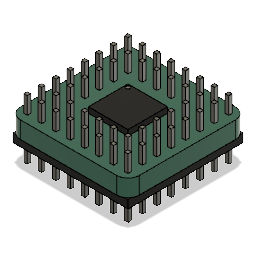
PGA2040 (Autodesk Fusion 360 design; units mm, degrees)
Autodesk Fusion 360 part; units mm, degrees
note: some values were not read from the file. Set by a fixed rule: which sketch regions a step uses.
sketch "Sketch1" plane through (0, 0, 0) normal (0, 1, 0) x (1, 0, 0)
  line L0 (-10.5, 10.5) -> (10.5, 10.5)
  line L1 (10.5, 10.5) -> (10.5, -10.5)
  line L2 (10.5, -10.5) -> (-10.5, -10.5)
  line L3 (-10.5, -10.5) -> (-10.5, 10.5)
  line L4 (-3.5, 3.5) -> (3.5, 3.5)
  line L5 (3.5, 3.5) -> (3.5, -3.5)
  line L6 (3.5, -3.5) -> (-3.5, -3.5)
  line L7 (-3.5, -3.5) -> (-3.5, 3.5)
  line L8 (-10.5, 8.89) -> (10.5, 8.89) construction
  line L9 (-8.89, 10.5) -> (-8.89, -10.5) construction
  line L10 (-10.5, -8.89) -> (10.5, -8.89) construction
  line L11 (8.89, 10.5) -> (8.89, -10.5) construction
  line L12 (-8.57, 8.57) -> (-9.21, 8.57)
  line L13 (-9.21, 8.57) -> (-9.21, 9.21)
  line L14 (-9.21, 9.21) -> (-8.57, 9.21)
  line L15 (-8.57, 9.21) -> (-8.57, 8.57)
  line L16 (-8.57, 8.57) -> (-9.21, 9.21) construction
  line L17 (-9.21, 8.57) -> (-8.57, 9.21) construction
  line L18 (-6.67, 9.21) -> (-6.03, 9.21)
  line L19 (-6.67, 8.57) -> (-6.67, 9.21)
  line L20 (-6.03, 8.57) -> (-6.67, 8.57)
  line L21 (-6.03, 9.21) -> (-6.03, 8.57)
  line L22 (-4.13, 9.21) -> (-3.49, 9.21)
  line L23 (-4.13, 8.57) -> (-4.13, 9.21)
  line L24 (-3.49, 8.57) -> (-4.13, 8.57)
  line L25 (-3.49, 9.21) -> (-3.49, 8.57)
  line L26 (-1.59, 9.21) -> (-0.95, 9.21)
  line L27 (-1.59, 8.57) -> (-1.59, 9.21)
  line L28 (-0.95, 8.57) -> (-1.59, 8.57)
  line L29 (-0.95, 9.21) -> (-0.95, 8.57)
  line L30 (0.95, 9.21) -> (1.59, 9.21)
  line L31 (0.95, 8.57) -> (0.95, 9.21)
  line L32 (1.59, 8.57) -> (0.95, 8.57)
  line L33 (1.59, 9.21) -> (1.59, 8.57)
  line L34 (3.49, 9.21) -> (4.13, 9.21)
  line L35 (3.49, 8.57) -> (3.49, 9.21)
  line L36 (4.13, 8.57) -> (3.49, 8.57)
  line L37 (4.13, 9.21) -> (4.13, 8.57)
  line L38 (6.03, 9.21) -> (6.67, 9.21)
  line L39 (6.03, 8.57) -> (6.03, 9.21)
  line L40 (6.67, 8.57) -> (6.03, 8.57)
  line L41 (6.67, 9.21) -> (6.67, 8.57)
  line L42 (8.57, 9.21) -> (9.21, 9.21)
  line L43 (8.57, 8.57) -> (8.57, 9.21)
  line L44 (9.21, 8.57) -> (8.57, 8.57)
  line L45 (9.21, 9.21) -> (9.21, 8.57)
  line L46 (-9.21, 6.67) -> (-8.57, 6.67)
  line L47 (-9.21, 6.03) -> (-9.21, 6.67)
  line L48 (-8.57, 6.03) -> (-9.21, 6.03)
  line L49 (-8.57, 6.67) -> (-8.57, 6.03)
  line L50 (-6.67, 6.67) -> (-6.03, 6.67)
  line L51 (-6.67, 6.03) -> (-6.67, 6.67)
  line L52 (-6.03, 6.03) -> (-6.67, 6.03)
  line L53 (-6.03, 6.67) -> (-6.03, 6.03)
  line L54 (-4.13, 6.67) -> (-3.49, 6.67)
  line L55 (-4.13, 6.03) -> (-4.13, 6.67)
  line L56 (-3.49, 6.03) -> (-4.13, 6.03)
  line L57 (-3.49, 6.67) -> (-3.49, 6.03)
  line L58 (-1.59, 6.67) -> (-0.95, 6.67)
  line L59 (-1.59, 6.03) -> (-1.59, 6.67)
  line L60 (-0.95, 6.03) -> (-1.59, 6.03)
  line L61 (-0.95, 6.67) -> (-0.95, 6.03)
  line L62 (0.95, 6.67) -> (1.59, 6.67)
  line L63 (0.95, 6.03) -> (0.95, 6.67)
  line L64 (1.59, 6.03) -> (0.95, 6.03)
  line L65 (1.59, 6.67) -> (1.59, 6.03)
  line L66 (3.49, 6.67) -> (4.13, 6.67)
  line L67 (3.49, 6.03) -> (3.49, 6.67)
  line L68 (4.13, 6.03) -> (3.49, 6.03)
  line L69 (4.13, 6.67) -> (4.13, 6.03)
  line L70 (6.03, 6.67) -> (6.67, 6.67)
  line L71 (6.03, 6.03) -> (6.03, 6.67)
  line L72 (6.67, 6.03) -> (6.03, 6.03)
  line L73 (6.67, 6.67) -> (6.67, 6.03)
  line L74 (8.57, 6.67) -> (9.21, 6.67)
  line L75 (8.57, 6.03) -> (8.57, 6.67)
  line L76 (9.21, 6.03) -> (8.57, 6.03)
  line L77 (9.21, 6.67) -> (9.21, 6.03)
  line L78 (-9.21, 4.13) -> (-8.57, 4.13)
  line L79 (-9.21, 3.49) -> (-9.21, 4.13)
  line L80 (-8.57, 3.49) -> (-9.21, 3.49)
  line L81 (-8.57, 4.13) -> (-8.57, 3.49)
  line L82 (-6.67, 4.13) -> (-6.03, 4.13)
  line L83 (-6.67, 3.49) -> (-6.67, 4.13)
  line L84 (-6.03, 3.49) -> (-6.67, 3.49)
  line L85 (-6.03, 4.13) -> (-6.03, 3.49)
  line L86 (6.03, 4.13) -> (6.67, 4.13)
  line L87 (6.03, 3.49) -> (6.03, 4.13)
  line L88 (6.67, 3.49) -> (6.03, 3.49)
  line L89 (6.67, 4.13) -> (6.67, 3.49)
  line L90 (8.57, 4.13) -> (9.21, 4.13)
  line L91 (8.57, 3.49) -> (8.57, 4.13)
  line L92 (9.21, 3.49) -> (8.57, 3.49)
  line L93 (9.21, 4.13) -> (9.21, 3.49)
  line L94 (-9.21, 1.59) -> (-8.57, 1.59)
  line L95 (-9.21, 0.95) -> (-9.21, 1.59)
  line L96 (-8.57, 0.95) -> (-9.21, 0.95)
  line L97 (-8.57, 1.59) -> (-8.57, 0.95)
  line L98 (-6.67, 1.59) -> (-6.03, 1.59)
  line L99 (-6.67, 0.95) -> (-6.67, 1.59)
  line L100 (-6.03, 0.95) -> (-6.67, 0.95)
  line L101 (-6.03, 1.59) -> (-6.03, 0.95)
  line L102 (6.03, 1.59) -> (6.67, 1.59)
  line L103 (6.03, 0.95) -> (6.03, 1.59)
  line L104 (6.67, 0.95) -> (6.03, 0.95)
  line L105 (6.67, 1.59) -> (6.67, 0.95)
  line L106 (8.57, 1.59) -> (9.21, 1.59)
  line L107 (8.57, 0.95) -> (8.57, 1.59)
  line L108 (9.21, 0.95) -> (8.57, 0.95)
  line L109 (9.21, 1.59) -> (9.21, 0.95)
  line L110 (-9.21, -0.95) -> (-8.57, -0.95)
  line L111 (-9.21, -1.59) -> (-9.21, -0.95)
  line L112 (-8.57, -1.59) -> (-9.21, -1.59)
  line L113 (-8.57, -0.95) -> (-8.57, -1.59)
  line L114 (-6.67, -0.95) -> (-6.03, -0.95)
  line L115 (-6.67, -1.59) -> (-6.67, -0.95)
  line L116 (-6.03, -1.59) -> (-6.67, -1.59)
  line L117 (-6.03, -0.95) -> (-6.03, -1.59)
  line L118 (6.03, -0.95) -> (6.67, -0.95)
  line L119 (6.03, -1.59) -> (6.03, -0.95)
  line L120 (6.67, -1.59) -> (6.03, -1.59)
  line L121 (6.67, -0.95) -> (6.67, -1.59)
  line L122 (8.57, -0.95) -> (9.21, -0.95)
  line L123 (8.57, -1.59) -> (8.57, -0.95)
  line L124 (9.21, -1.59) -> (8.57, -1.59)
  line L125 (9.21, -0.95) -> (9.21, -1.59)
  line L126 (-9.21, -3.49) -> (-8.57, -3.49)
  line L127 (-9.21, -4.13) -> (-9.21, -3.49)
  line L128 (-8.57, -4.13) -> (-9.21, -4.13)
  line L129 (-8.57, -3.49) -> (-8.57, -4.13)
  line L130 (-6.67, -3.49) -> (-6.03, -3.49)
  line L131 (-6.67, -4.13) -> (-6.67, -3.49)
  line L132 (-6.03, -4.13) -> (-6.67, -4.13)
  line L133 (-6.03, -3.49) -> (-6.03, -4.13)
  line L134 (6.03, -3.49) -> (6.67, -3.49)
  line L135 (6.03, -4.13) -> (6.03, -3.49)
  line L136 (6.67, -4.13) -> (6.03, -4.13)
  line L137 (6.67, -3.49) -> (6.67, -4.13)
  line L138 (8.57, -3.49) -> (9.21, -3.49)
  line L139 (8.57, -4.13) -> (8.57, -3.49)
  line L140 (9.21, -4.13) -> (8.57, -4.13)
  line L141 (9.21, -3.49) -> (9.21, -4.13)
  line L142 (-9.21, -6.03) -> (-8.57, -6.03)
  line L143 (-9.21, -6.67) -> (-9.21, -6.03)
  line L144 (-8.57, -6.67) -> (-9.21, -6.67)
  line L145 (-8.57, -6.03) -> (-8.57, -6.67)
  line L146 (-6.67, -6.03) -> (-6.03, -6.03)
  line L147 (-6.67, -6.67) -> (-6.67, -6.03)
  line L148 (-6.03, -6.67) -> (-6.67, -6.67)
  line L149 (-6.03, -6.03) -> (-6.03, -6.67)
  line L150 (-4.13, -6.03) -> (-3.49, -6.03)
  line L151 (-4.13, -6.67) -> (-4.13, -6.03)
  line L152 (-3.49, -6.67) -> (-4.13, -6.67)
  line L153 (-3.49, -6.03) -> (-3.49, -6.67)
  line L154 (-1.59, -6.03) -> (-0.95, -6.03)
  line L155 (-1.59, -6.67) -> (-1.59, -6.03)
  line L156 (-0.95, -6.67) -> (-1.59, -6.67)
  line L157 (-0.95, -6.03) -> (-0.95, -6.67)
  line L158 (0.95, -6.03) -> (1.59, -6.03)
  line L159 (0.95, -6.67) -> (0.95, -6.03)
  line L160 (1.59, -6.67) -> (0.95, -6.67)
  line L161 (1.59, -6.03) -> (1.59, -6.67)
  line L162 (3.49, -6.03) -> (4.13, -6.03)
  line L163 (3.49, -6.67) -> (3.49, -6.03)
  line L164 (4.13, -6.67) -> (3.49, -6.67)
  line L165 (4.13, -6.03) -> (4.13, -6.67)
  line L166 (6.03, -6.03) -> (6.67, -6.03)
  line L167 (6.03, -6.67) -> (6.03, -6.03)
  line L168 (6.67, -6.67) -> (6.03, -6.67)
  line L169 (6.67, -6.03) -> (6.67, -6.67)
  line L170 (8.57, -6.03) -> (9.21, -6.03)
  line L171 (8.57, -6.67) -> (8.57, -6.03)
  line L172 (9.21, -6.67) -> (8.57, -6.67)
  line L173 (9.21, -6.03) -> (9.21, -6.67)
  line L174 (-9.21, -8.57) -> (-8.57, -8.57)
  line L175 (-9.21, -9.21) -> (-9.21, -8.57)
  line L176 (-8.57, -9.21) -> (-9.21, -9.21)
  line L177 (-8.57, -8.57) -> (-8.57, -9.21)
  line L178 (-6.67, -8.57) -> (-6.03, -8.57)
  line L179 (-6.67, -9.21) -> (-6.67, -8.57)
  line L180 (-6.03, -9.21) -> (-6.67, -9.21)
  line L181 (-6.03, -8.57) -> (-6.03, -9.21)
  line L182 (-4.13, -8.57) -> (-3.49, -8.57)
  line L183 (-4.13, -9.21) -> (-4.13, -8.57)
  line L184 (-3.49, -9.21) -> (-4.13, -9.21)
  line L185 (-3.49, -8.57) -> (-3.49, -9.21)
  line L186 (-1.59, -8.57) -> (-0.95, -8.57)
  line L187 (-1.59, -9.21) -> (-1.59, -8.57)
  line L188 (-0.95, -9.21) -> (-1.59, -9.21)
  line L189 (-0.95, -8.57) -> (-0.95, -9.21)
  line L190 (0.95, -8.57) -> (1.59, -8.57)
  line L191 (0.95, -9.21) -> (0.95, -8.57)
  line L192 (1.59, -9.21) -> (0.95, -9.21)
  line L193 (1.59, -8.57) -> (1.59, -9.21)
  line L194 (3.49, -8.57) -> (4.13, -8.57)
  line L195 (3.49, -9.21) -> (3.49, -8.57)
  line L196 (4.13, -9.21) -> (3.49, -9.21)
  line L197 (4.13, -8.57) -> (4.13, -9.21)
  line L198 (6.03, -8.57) -> (6.67, -8.57)
  line L199 (6.03, -9.21) -> (6.03, -8.57)
  line L200 (6.67, -9.21) -> (6.03, -9.21)
  line L201 (6.67, -8.57) -> (6.67, -9.21)
  line L202 (8.57, -8.57) -> (9.21, -8.57)
  line L203 (8.57, -9.21) -> (8.57, -8.57)
  line L204 (9.21, -9.21) -> (8.57, -9.21)
  line L205 (9.21, -8.57) -> (9.21, -9.21)
  circle A0 centre (-3, 3) radius 0.375
  point P0 (-8.89, 8.89)
  dimension "d1" = 10.5
  dimension "d2" = 21
  dimension "d3" = 10.5
  dimension "d4" = 21
  dimension "d5" = 7
  dimension "d6" = 7
  dimension "d7" = 3.5
  dimension "d8" = 3.5
  dimension "d20" = 17.78
  dimension "d21" = 17.78
  dimension "d22" = 8.89
  dimension "d23" = 8.89
  dimension "d38" = 0.64
  dimension "d39" = 0.64
  dimension "d46" = 2.54
  dimension "d47" = -2.54
  dimension "d52" = 0.5
  dimension "d53" = 0.5
  dimension "d54" = 0.75
  constraint horizontal L0
  constraint vertical L1
  constraint horizontal L2
  constraint vertical L3
  constraint horizontal L4
  constraint vertical L5
  constraint horizontal L6
  constraint vertical L7
  constraint perpendicular L1 L8
  constraint coincident L1 L8.end
  constraint coincident L3 L8.start
  constraint perpendicular L2 L9
  constraint coincident L2 L9.end
  constraint coincident L0 L9.start
  constraint parallel L2 L10
  constraint coincident L1 L10.end
  constraint coincident L3 L10.start
  constraint perpendicular L2 L11
  constraint coincident L2 L11.end
  constraint coincident L0 L11.start
  constraint horizontal L12
  constraint perpendicular L12 L13
  constraint parallel L12 L14
  constraint parallel L13 L15
  constraint coincident L16 P0
  constraint coincident L17 P0
  constraint coincident L9 P0
  constraint coincident L8 P0
  measures "d1" distance of origin L0
  measures "d2" distance of L0 L2
  measures "d3" distance of origin L3
  measures "d4" distance of L1 L3
  measures "d5" distance of L4.start L4.end
  measures "d6" distance of L4.start L6.end
  measures "d7" distance of origin L4
  measures "d8" distance of origin L7
  measures "d20" distance of L9 L11
  measures "d21" distance of L8 L10
  measures "d22" distance of origin L10
  measures "d23" distance of origin L11
  measures "d38" distance of L13.end L14.end
  measures "d39" distance of L12.start L14.end
  measures "d52" distance of L7 A0.centre
  measures "d53" vertical distance of L4.start A0.centre
  measures "d54" diameter of A0
extrude "Extrude1" add sketch "Sketch1" along normal blind 1 contours L4 L5 L6 L7 | A0
extrude "Extrude2" add sketch "Sketch1" against normal blind 3 contours L0 L1 L2 L3 | L4 L5 L6 L7 | L12 L13 L14 L15 | L18 L19 L20 L21 | L22 L23 L24 L25 | L26 L27 L28 L29 | L30 L31 L32 L33 | L34 L35 L36 L37 | L38 L39 L40 L41 | L42 L43 L44 L45 | L46 L47 L48 L49 | L50 L51 L52 L53 | L54 L55 L56 L57 | L58 L59 L60 L61 | L62 L63 L64 L65 | L66 L67 L68 L69 | L70 L71 L72 L73 | L74 L75 L76 L77 | L78 L79 L80 L81 | L82 L83 L84 L85 | L86 L87 L88 L89 | L90 L91 L92 L93 | L94 L95 L96 L97 | L98 L99 L100 L101 | L102 L103 L104 L105 | L106 L107 L108 L109 | L110 L111 L112 L113 | L114 L115 L116 L117 | L118 L119 L120 L121 | L122 L123 L124 L125 | L126 L127 L128 L129 | L130 L131 L132 L133 | L134 L135 L136 L137 | L138 L139 L140 L141 | L142 L143 L144 L145 | L146 L147 L148 L149 | L150 L151 L152 L153 | L154 L155 L156 L157 | L158 L159 L160 L161 | L162 L163 L164 L165 | L166 L167 L168 L169 | L170 L171 L172 L173 | L174 L175 L176 L177 | L178 L179 L180 L181 | L182 L183 L184 L185 | L186 L187 L188 L189 | L190 L191 L192 L193 | L194 L195 L196 L197 | L198 L199 L200 L201 | L202 L203 L204 L205 | A0
extrude "Extrude3" add sketch "Sketch1" along normal blind 3 and the other way blind 7.5 contours L12 L13 L14 L15 | L18 L19 L20 L21 | L22 L23 L24 L25 | L26 L27 L28 L29 | L30 L31 L32 L33 | L34 L35 L36 L37 | L38 L39 L40 L41 | L42 L43 L44 L45 | L46 L47 L48 L49 | L50 L51 L52 L53 | L54 L55 L56 L57 | L58 L59 L60 L61 | L62 L63 L64 L65 | L66 L67 L68 L69 | L70 L71 L72 L73 | L74 L75 L76 L77 | L78 L79 L80 L81 | L82 L83 L84 L85 | L86 L87 L88 L89 | L90 L91 L92 L93 | L94 L95 L96 L97 | L98 L99 L100 L101 | L102 L103 L104 L105 | L106 L107 L108 L109 | L110 L111 L112 L113 | L114 L115 L116 L117 | L118 L119 L120 L121 | L122 L123 L124 L125 | L126 L127 L128 L129 | L130 L131 L132 L133 | L134 L135 L136 L137 | L138 L139 L140 L141 | L142 L143 L144 L145 | L146 L147 L148 L149 | L150 L151 L152 L153 | L154 L155 L156 L157 | L158 L159 L160 L161 | L162 L163 L164 L165 | L166 L167 L168 L169 | L170 L171 L172 L173 | L174 L175 L176 L177 | L178 L179 L180 L181 | L182 L183 L184 L185 | L186 L187 L188 L189 | L190 L191 L192 L193 | L194 L195 L196 L197 | L198 L199 L200 L201 | L202 L203 L204 L205
extrude "Extrude4" cut sketch "Sketch1" against normal blind 0.1 from surface at 1 contours A0
sketch "Sketch2" plane through (0, -3, 0) normal (0, -1, 0) x (1, 0, 0)
  line L0 (10.5, -10.5) -> (10.5, 10.5)
  line L1 (10.5, 10.5) -> (-10.5, 10.5)
  line L2 (-10.5, 10.5) -> (-10.5, -10.5)
  line L3 (-10.5, -10.5) -> (10.5, -10.5)
  line L4 (6.67, -0.95) -> (6.67, -1.59)
  line L5 (6.67, -1.59) -> (6.03, -1.59)
  line L6 (6.03, -1.59) -> (6.03, -0.95)
  line L7 (6.03, -0.95) -> (6.67, -0.95)
  line L8 (9.21, -3.49) -> (9.21, -4.13)
  line L9 (9.21, -4.13) -> (8.57, -4.13)
  line L10 (8.57, -4.13) -> (8.57, -3.49)
  line L11 (8.57, -3.49) -> (9.21, -3.49)
  line L12 (9.21, -8.57) -> (9.21, -9.21)
  line L13 (9.21, -9.21) -> (8.57, -9.21)
  line L14 (8.57, -9.21) -> (8.57, -8.57)
  line L15 (8.57, -8.57) -> (9.21, -8.57)
  line L16 (1.59, -6.03) -> (1.59, -6.67)
  line L17 (1.59, -6.67) -> (0.95, -6.67)
  line L18 (0.95, -6.67) -> (0.95, -6.03)
  line L19 (0.95, -6.03) -> (1.59, -6.03)
  line L20 (9.21, 4.13) -> (9.21, 3.49)
  line L21 (9.21, 3.49) -> (8.57, 3.49)
  line L22 (8.57, 3.49) -> (8.57, 4.13)
  line L23 (8.57, 4.13) -> (9.21, 4.13)
  line L24 (9.21, 9.21) -> (9.21, 8.57)
  line L25 (9.21, 8.57) -> (8.57, 8.57)
  line L26 (8.57, 8.57) -> (8.57, 9.21)
  line L27 (8.57, 9.21) -> (9.21, 9.21)
  line L28 (1.59, 6.67) -> (1.59, 6.03)
  line L29 (1.59, 6.03) -> (0.95, 6.03)
  line L30 (0.95, 6.03) -> (0.95, 6.67)
  line L31 (0.95, 6.67) -> (1.59, 6.67)
  line L32 (-3.49, 9.21) -> (-3.49, 8.57)
  line L33 (-3.49, 8.57) -> (-4.13, 8.57)
  line L34 (-4.13, 8.57) -> (-4.13, 9.21)
  line L35 (-4.13, 9.21) -> (-3.49, 9.21)
  line L36 (-6.03, -8.57) -> (-6.03, -9.21)
  line L37 (-6.03, -9.21) -> (-6.67, -9.21)
  line L38 (-6.67, -9.21) -> (-6.67, -8.57)
  line L39 (-6.67, -8.57) -> (-6.03, -8.57)
  line L40 (-6.03, 1.59) -> (-6.03, 0.95)
  line L41 (-6.03, 0.95) -> (-6.67, 0.95)
  line L42 (-6.67, 0.95) -> (-6.67, 1.59)
  line L43 (-6.67, 1.59) -> (-6.03, 1.59)
  line L44 (-8.57, 9.21) -> (-8.57, 8.57)
  line L45 (-8.57, 8.57) -> (-9.21, 8.57)
  line L46 (-9.21, 8.57) -> (-9.21, 9.21)
  line L47 (-9.21, 9.21) -> (-8.57, 9.21)
  line L48 (-8.57, -0.95) -> (-8.57, -1.59)
  line L49 (-8.57, -1.59) -> (-9.21, -1.59)
  line L50 (-9.21, -1.59) -> (-9.21, -0.95)
  line L51 (-9.21, -0.95) -> (-8.57, -0.95)
  line L52 (-8.57, -8.57) -> (-8.57, -9.21)
  line L53 (-8.57, -9.21) -> (-9.21, -9.21)
  line L54 (-9.21, -9.21) -> (-9.21, -8.57)
  line L55 (-9.21, -8.57) -> (-8.57, -8.57)
  line L56 (-8.57, 1.59) -> (-8.57, 0.95)
  line L57 (-8.57, 0.95) -> (-9.21, 0.95)
  line L58 (-9.21, 0.95) -> (-9.21, 1.59)
  line L59 (-9.21, 1.59) -> (-8.57, 1.59)
  line L60 (-6.03, 9.21) -> (-6.03, 8.57)
  line L61 (-6.03, 8.57) -> (-6.67, 8.57)
  line L62 (-6.67, 8.57) -> (-6.67, 9.21)
  line L63 (-6.67, 9.21) -> (-6.03, 9.21)
  line L64 (-6.03, -0.95) -> (-6.03, -1.59)
  line L65 (-6.03, -1.59) -> (-6.67, -1.59)
  line L66 (-6.67, -1.59) -> (-6.67, -0.95)
  line L67 (-6.67, -0.95) -> (-6.03, -0.95)
  line L68 (-3.49, -8.57) -> (-3.49, -9.21)
  line L69 (-3.49, -9.21) -> (-4.13, -9.21)
  line L70 (-4.13, -9.21) -> (-4.13, -8.57)
  line L71 (-4.13, -8.57) -> (-3.49, -8.57)
  line L72 (-0.95, 9.21) -> (-0.95, 8.57)
  line L73 (-0.95, 8.57) -> (-1.59, 8.57)
  line L74 (-1.59, 8.57) -> (-1.59, 9.21)
  line L75 (-1.59, 9.21) -> (-0.95, 9.21)
  line L76 (4.13, 6.67) -> (4.13, 6.03)
  line L77 (4.13, 6.03) -> (3.49, 6.03)
  line L78 (3.49, 6.03) -> (3.49, 6.67)
  line L79 (3.49, 6.67) -> (4.13, 6.67)
  line L80 (6.67, 6.67) -> (6.67, 6.03)
  line L81 (6.67, 6.03) -> (6.03, 6.03)
  line L82 (6.03, 6.03) -> (6.03, 6.67)
  line L83 (6.03, 6.67) -> (6.67, 6.67)
  line L84 (-0.95, -6.03) -> (-0.95, -6.67)
  line L85 (-0.95, -6.67) -> (-1.59, -6.67)
  line L86 (-1.59, -6.67) -> (-1.59, -6.03)
  line L87 (-1.59, -6.03) -> (-0.95, -6.03)
  line L88 (4.13, -6.03) -> (4.13, -6.67)
  line L89 (4.13, -6.67) -> (3.49, -6.67)
  line L90 (3.49, -6.67) -> (3.49, -6.03)
  line L91 (3.49, -6.03) -> (4.13, -6.03)
  line L92 (9.21, -6.03) -> (9.21, -6.67)
  line L93 (9.21, -6.67) -> (8.57, -6.67)
  line L94 (8.57, -6.67) -> (8.57, -6.03)
  line L95 (8.57, -6.03) -> (9.21, -6.03)
  line L96 (9.21, -0.95) -> (9.21, -1.59)
  line L97 (9.21, -1.59) -> (8.57, -1.59)
  line L98 (8.57, -1.59) -> (8.57, -0.95)
  line L99 (8.57, -0.95) -> (9.21, -0.95)
  line L100 (6.67, 1.59) -> (6.67, 0.95)
  line L101 (6.67, 0.95) -> (6.03, 0.95)
  line L102 (6.03, 0.95) -> (6.03, 1.59)
  line L103 (6.03, 1.59) -> (6.67, 1.59)
  line L104 (6.67, -3.49) -> (6.67, -4.13)
  line L105 (6.67, -4.13) -> (6.03, -4.13)
  line L106 (6.03, -4.13) -> (6.03, -3.49)
  line L107 (6.03, -3.49) -> (6.67, -3.49)
  line L108 (6.67, -8.57) -> (6.67, -9.21)
  line L109 (6.67, -9.21) -> (6.03, -9.21)
  line L110 (6.03, -9.21) -> (6.03, -8.57)
  line L111 (6.03, -8.57) -> (6.67, -8.57)
  line L112 (1.59, -8.57) -> (1.59, -9.21)
  line L113 (1.59, -9.21) -> (0.95, -9.21)
  line L114 (0.95, -9.21) -> (0.95, -8.57)
  line L115 (0.95, -8.57) -> (1.59, -8.57)
  line L116 (6.67, 4.13) -> (6.67, 3.49)
  line L117 (6.67, 3.49) -> (6.03, 3.49)
  line L118 (6.03, 3.49) -> (6.03, 4.13)
  line L119 (6.03, 4.13) -> (6.67, 4.13)
  line L120 (6.67, 9.21) -> (6.67, 8.57)
  line L121 (6.67, 8.57) -> (6.03, 8.57)
  line L122 (6.03, 8.57) -> (6.03, 9.21)
  line L123 (6.03, 9.21) -> (6.67, 9.21)
  line L124 (1.59, 9.21) -> (1.59, 8.57)
  line L125 (1.59, 8.57) -> (0.95, 8.57)
  line L126 (0.95, 8.57) -> (0.95, 9.21)
  line L127 (0.95, 9.21) -> (1.59, 9.21)
  line L128 (-3.49, 6.67) -> (-3.49, 6.03)
  line L129 (-3.49, 6.03) -> (-4.13, 6.03)
  line L130 (-4.13, 6.03) -> (-4.13, 6.67)
  line L131 (-4.13, 6.67) -> (-3.49, 6.67)
  line L132 (-6.03, -6.03) -> (-6.03, -6.67)
  line L133 (-6.03, -6.67) -> (-6.67, -6.67)
  line L134 (-6.67, -6.67) -> (-6.67, -6.03)
  line L135 (-6.67, -6.03) -> (-6.03, -6.03)
  line L136 (-6.03, 4.13) -> (-6.03, 3.49)
  line L137 (-6.03, 3.49) -> (-6.67, 3.49)
  line L138 (-6.67, 3.49) -> (-6.67, 4.13)
  line L139 (-6.67, 4.13) -> (-6.03, 4.13)
  line L140 (-8.57, 6.67) -> (-8.57, 6.03)
  line L141 (-8.57, 6.03) -> (-9.21, 6.03)
  line L142 (-9.21, 6.03) -> (-9.21, 6.67)
  line L143 (-9.21, 6.67) -> (-8.57, 6.67)
  line L144 (-8.57, -3.49) -> (-8.57, -4.13)
  line L145 (-8.57, -4.13) -> (-9.21, -4.13)
  line L146 (-9.21, -4.13) -> (-9.21, -3.49)
  line L147 (-9.21, -3.49) -> (-8.57, -3.49)
  line L148 (-8.57, -6.03) -> (-8.57, -6.67)
  line L149 (-8.57, -6.67) -> (-9.21, -6.67)
  line L150 (-9.21, -6.67) -> (-9.21, -6.03)
  line L151 (-9.21, -6.03) -> (-8.57, -6.03)
  line L152 (-8.57, 4.13) -> (-8.57, 3.49)
  line L153 (-8.57, 3.49) -> (-9.21, 3.49)
  line L154 (-9.21, 3.49) -> (-9.21, 4.13)
  line L155 (-9.21, 4.13) -> (-8.57, 4.13)
  line L156 (-6.03, 6.67) -> (-6.03, 6.03)
  line L157 (-6.03, 6.03) -> (-6.67, 6.03)
  line L158 (-6.67, 6.03) -> (-6.67, 6.67)
  line L159 (-6.67, 6.67) -> (-6.03, 6.67)
  line L160 (-6.03, -3.49) -> (-6.03, -4.13)
  line L161 (-6.03, -4.13) -> (-6.67, -4.13)
  line L162 (-6.67, -4.13) -> (-6.67, -3.49)
  line L163 (-6.67, -3.49) -> (-6.03, -3.49)
  line L164 (-3.49, -6.03) -> (-3.49, -6.67)
  line L165 (-3.49, -6.67) -> (-4.13, -6.67)
  line L166 (-4.13, -6.67) -> (-4.13, -6.03)
  line L167 (-4.13, -6.03) -> (-3.49, -6.03)
  line L168 (-0.95, 6.67) -> (-0.95, 6.03)
  line L169 (-0.95, 6.03) -> (-1.59, 6.03)
  line L170 (-1.59, 6.03) -> (-1.59, 6.67)
  line L171 (-1.59, 6.67) -> (-0.95, 6.67)
  line L172 (4.13, 9.21) -> (4.13, 8.57)
  line L173 (4.13, 8.57) -> (3.49, 8.57)
  line L174 (3.49, 8.57) -> (3.49, 9.21)
  line L175 (3.49, 9.21) -> (4.13, 9.21)
  line L176 (9.21, 6.67) -> (9.21, 6.03)
  line L177 (9.21, 6.03) -> (8.57, 6.03)
  line L178 (8.57, 6.03) -> (8.57, 6.67)
  line L179 (8.57, 6.67) -> (9.21, 6.67)
  line L180 (-0.95, -8.57) -> (-0.95, -9.21)
  line L181 (-0.95, -9.21) -> (-1.59, -9.21)
  line L182 (-1.59, -9.21) -> (-1.59, -8.57)
  line L183 (-1.59, -8.57) -> (-0.95, -8.57)
  line L184 (4.13, -8.57) -> (4.13, -9.21)
  line L185 (4.13, -9.21) -> (3.49, -9.21)
  line L186 (3.49, -9.21) -> (3.49, -8.57)
  line L187 (3.49, -8.57) -> (4.13, -8.57)
  line L188 (6.67, -6.03) -> (6.67, -6.67)
  line L189 (6.67, -6.67) -> (6.03, -6.67)
  line L190 (6.03, -6.67) -> (6.03, -6.03)
  line L191 (6.03, -6.03) -> (6.67, -6.03)
  line L192 (9.21, 1.59) -> (9.21, 0.95)
  line L193 (9.21, 0.95) -> (8.57, 0.95)
  line L194 (8.57, 0.95) -> (8.57, 1.59)
  line L195 (8.57, 1.59) -> (9.21, 1.59)
  line L196 (10.16, 10.16) -> (-10.16, 10.16)
  line L197 (-10.16, 10.16) -> (-10.16, -10.16)
  line L198 (-10.16, -10.16) -> (10.16, -10.16)
  line L199 (10.16, -10.16) -> (10.16, 10.16)
  line L200 (-5.16, 5.16) -> (5.16, 5.16)
  line L201 (5.16, 5.16) -> (5.16, -5.16)
  line L202 (5.16, -5.16) -> (-5.16, -5.16)
  line L203 (-5.16, -5.16) -> (-5.16, 5.16)
  dimension "d60" = 5
  dimension "d61" = 5
  dimension "d62" = 5
  dimension "d63" = 5
  dimension "d64" = 20.32
  dimension "d65" = 20.32
  dimension "d66" = 10.16
  dimension "d68" = 10.16
  constraint horizontal L196
  constraint vertical L197
  constraint horizontal L198
  constraint vertical L199
  constraint horizontal L200
  constraint vertical L201
  constraint horizontal L202
  constraint vertical L203
  measures "d60" distance of L199 L201
  measures "d61" distance of L196 L200
  measures "d62" distance of L197 L203
  measures "d63" distance of L198 L202
  measures "d64" distance of L196.start L196.end
  measures "d65" distance of L196.start L198.end
  measures "d66" distance of origin L199
  measures "d68" distance of origin L196
fillet "Fillet1" radius 2 3 edges at (-10.5, -1.5, 10.5) (10.5, -1.5, 10.5) (10.5, -1.5, -10.5)
extrude "Extrude5" add sketch "Sketch2" along normal blind 1.5 contours L196 L197 L198 L199
equation "d1 = d2 / 2"
equation "d3 = d1"
equation "d4 = d2"
equation "d5 = d6"
equation "d7 = d6 / 2"
equation "d8 = d7"
equation "d14 = 2.54 mm"
equation "d16 = d14"
equation "d17 = d16"
equation "d18 = d17 * 4"
equation "d20 = d16 * 7"
equation "d21 = d20"
equation "d22 = d21 / 2"
equation "d23 = d20 / 2"
equation "d24 = 0.64 mm"
equation "d25 = d24"
equation "d28 = d16"
equation "d29 = d28"
equation "d30 = d29"
equation "d39 = d38"
equation "d53 = d52"
equation "d61 = d60"
equation "d62 = d61"
equation "d63 = d60"
equation "d64 = ( 8 * 2.54 ) * 1 mm"
equation "d65 = d64"
equation "d66 = d64 / 2"
equation "d68 = d66"
named bodies: "rp2040"
